Autodesk Inventor part; units mm, degrees
(part 10 of 13)
  arc A3550 (1.0789, 34.461) -> (1.0789, 34.335) centre (1.0789, 34.398) ccw
  line L3551 (3.0258, 34.335) -> (6.4346, 34.335)
  arc A3551 (6.4346, 34.335) -> (6.4346, 34.461) centre (6.4346, 34.398) ccw
  line L3552 (6.4346, 34.461) -> (3.0258, 34.461)
  arc A3552 (3.0258, 34.461) -> (3.0258, 34.335) centre (3.0258, 34.398) ccw
  line L3553 (8.9653, 34.335) -> (17.121, 34.335)
  arc A3553 (17.121, 34.335) -> (17.121, 34.461) centre (17.121, 34.398) ccw
  line L3554 (17.121, 34.461) -> (8.9653, 34.461)
  arc A3554 (8.9653, 34.461) -> (8.9653, 34.335) centre (8.9653, 34.398) ccw
  line L3555 (1.0789, 34.461) -> (2.0784, 34.461)
  arc A3555 (2.0784, 34.461) -> (2.0784, 34.587) centre (2.0784, 34.524) ccw
  line L3556 (2.0784, 34.587) -> (1.0789, 34.587)
  arc A3556 (1.0789, 34.587) -> (1.0789, 34.461) centre (1.0789, 34.524) ccw
  line L3557 (2.7216, 34.461) -> (6.4346, 34.461)
  arc A3557 (6.4346, 34.461) -> (6.4346, 34.587) centre (6.4346, 34.524) ccw
  line L3558 (6.4346, 34.587) -> (2.7216, 34.587)
  arc A3558 (2.7216, 34.587) -> (2.7216, 34.461) centre (2.7216, 34.524) ccw
  line L3559 (8.9653, 34.461) -> (17.121, 34.461)
  arc A3559 (17.121, 34.461) -> (17.121, 34.587) centre (17.121, 34.524) ccw
  line L3560 (17.121, 34.587) -> (8.9653, 34.587)
  arc A3560 (8.9653, 34.587) -> (8.9653, 34.461) centre (8.9653, 34.524) ccw
  line L3561 (1.0789, 34.587) -> (6.4346, 34.587)
  arc A3561 (6.4346, 34.587) -> (6.4346, 34.713) centre (6.4346, 34.65) ccw
  line L3562 (6.4346, 34.713) -> (1.0789, 34.713)
  arc A3562 (1.0789, 34.713) -> (1.0789, 34.587) centre (1.0789, 34.65) ccw
  line L3563 (8.9653, 34.587) -> (17.121, 34.587)
  arc A3563 (17.121, 34.587) -> (17.121, 34.713) centre (17.121, 34.65) ccw
  line L3564 (17.121, 34.713) -> (8.9653, 34.713)
  arc A3564 (8.9653, 34.713) -> (8.9653, 34.587) centre (8.9653, 34.65) ccw
  line L3565 (1.0789, 34.713) -> (6.4346, 34.713)
  arc A3565 (6.4346, 34.713) -> (6.4346, 34.839) centre (6.4346, 34.776) ccw
  line L3566 (6.4346, 34.839) -> (1.0789, 34.839)
  arc A3566 (1.0789, 34.839) -> (1.0789, 34.713) centre (1.0789, 34.776) ccw
  line L3567 (8.9653, 34.713) -> (17.121, 34.713)
  arc A3567 (17.121, 34.713) -> (17.121, 34.839) centre (17.121, 34.776) ccw
  line L3568 (17.121, 34.839) -> (8.9653, 34.839)
  arc A3568 (8.9653, 34.839) -> (8.9653, 34.713) centre (8.9653, 34.776) ccw
  line L3569 (1.0789, 34.839) -> (6.4803, 34.839)
  arc A3569 (6.4803, 34.839) -> (6.4803, 34.965) centre (6.4803, 34.902) ccw
  line L3570 (6.4803, 34.965) -> (1.0789, 34.965)
  arc A3570 (1.0789, 34.965) -> (1.0789, 34.839) centre (1.0789, 34.902) ccw
  line L3571 (8.9197, 34.839) -> (17.121, 34.839)
  arc A3571 (17.121, 34.839) -> (17.121, 34.965) centre (17.121, 34.902) ccw
  line L3572 (17.121, 34.965) -> (8.9197, 34.965)
  arc A3572 (8.9197, 34.965) -> (8.9197, 34.839) centre (8.9197, 34.902) ccw
  line L3573 (1.0789, 34.965) -> (6.5325, 34.965)
  arc A3573 (6.5325, 34.965) -> (6.5325, 35.091) centre (6.5325, 35.028) ccw
  line L3574 (6.5325, 35.091) -> (1.0789, 35.091)
  arc A3574 (1.0789, 35.091) -> (1.0789, 34.965) centre (1.0789, 35.028) ccw
  line L3575 (8.8675, 34.965) -> (17.121, 34.965)
  arc A3575 (17.121, 34.965) -> (17.121, 35.091) centre (17.121, 35.028) ccw
  line L3576 (17.121, 35.091) -> (8.8675, 35.091)
  arc A3576 (8.8675, 35.091) -> (8.8675, 34.965) centre (8.8675, 35.028) ccw
  line L3577 (1.0789, 35.091) -> (6.5847, 35.091)
  arc A3577 (6.5847, 35.091) -> (6.5847, 35.217) centre (6.5847, 35.154) ccw
  line L3578 (6.5847, 35.217) -> (1.0789, 35.217)
  arc A3578 (1.0789, 35.217) -> (1.0789, 35.091) centre (1.0789, 35.154) ccw
  line L3579 (8.8153, 35.091) -> (17.121, 35.091)
  arc A3579 (17.121, 35.091) -> (17.121, 35.217) centre (17.121, 35.154) ccw
  line L3580 (17.121, 35.217) -> (8.8153, 35.217)
  arc A3580 (8.8153, 35.217) -> (8.8153, 35.091) centre (8.8153, 35.154) ccw
  line L3581 (1.0789, 35.217) -> (6.6505, 35.217)
  arc A3581 (6.6505, 35.217) -> (6.6505, 35.343) centre (6.6505, 35.28) ccw
  line L3582 (6.6505, 35.343) -> (1.0789, 35.343)
  arc A3582 (1.0789, 35.343) -> (1.0789, 35.217) centre (1.0789, 35.28) ccw
  line L3583 (8.7494, 35.217) -> (17.121, 35.217)
  arc A3583 (17.121, 35.217) -> (17.121, 35.343) centre (17.121, 35.28) ccw
  line L3584 (17.121, 35.343) -> (8.7494, 35.343)
  arc A3584 (8.7494, 35.343) -> (8.7494, 35.217) centre (8.7494, 35.28) ccw
  line L3585 (1.0789, 35.343) -> (6.7765, 35.343)
  arc A3585 (6.7765, 35.343) -> (6.7765, 35.469) centre (6.7765, 35.406) ccw
  line L3586 (6.7765, 35.469) -> (1.0789, 35.469)
  arc A3586 (1.0789, 35.469) -> (1.0789, 35.343) centre (1.0789, 35.406) ccw
  line L3587 (8.6234, 35.343) -> (17.121, 35.343)
  arc A3587 (17.121, 35.343) -> (17.121, 35.469) centre (17.121, 35.406) ccw
  line L3588 (17.121, 35.469) -> (8.6234, 35.469)
  arc A3588 (8.6234, 35.469) -> (8.6234, 35.343) centre (8.6234, 35.406) ccw
  line L3589 (1.0789, 35.469) -> (6.9025, 35.469)
  arc A3589 (6.9025, 35.469) -> (6.9025, 35.595) centre (6.9025, 35.532) ccw
  line L3590 (6.9025, 35.595) -> (1.0789, 35.595)
  arc A3590 (1.0789, 35.595) -> (1.0789, 35.469) centre (1.0789, 35.532) ccw
  line L3591 (8.4974, 35.469) -> (17.121, 35.469)
  arc A3591 (17.121, 35.469) -> (17.121, 35.595) centre (17.121, 35.532) ccw
  line L3592 (17.121, 35.595) -> (8.4974, 35.595)
  arc A3592 (8.4974, 35.595) -> (8.4974, 35.469) centre (8.4974, 35.532) ccw
  line L3593 (1.0789, 35.595) -> (7.0926, 35.595)
  arc A3593 (7.0926, 35.595) -> (7.0926, 35.721) centre (7.0926, 35.658) ccw
  line L3594 (7.0926, 35.721) -> (1.0789, 35.721)
  arc A3594 (1.0789, 35.721) -> (1.0789, 35.595) centre (1.0789, 35.658) ccw
  line L3595 (8.3074, 35.595) -> (17.121, 35.595)
  arc A3595 (17.121, 35.595) -> (17.121, 35.721) centre (17.121, 35.658) ccw
  line L3596 (17.121, 35.721) -> (8.3074, 35.721)
  arc A3596 (8.3074, 35.721) -> (8.3074, 35.595) centre (8.3074, 35.658) ccw
  line L3597 (1.0789, 35.721) -> (2.0347, 35.721)
  arc A3597 (2.0347, 35.721) -> (2.0347, 35.847) centre (2.0347, 35.784) ccw
  line L3598 (2.0347, 35.847) -> (1.0789, 35.847)
  arc A3598 (1.0789, 35.847) -> (1.0789, 35.721) centre (1.0789, 35.784) ccw
  line L3599 (2.337, 35.721) -> (2.4628, 35.721)
  arc A3599 (2.4628, 35.721) -> (2.4628, 35.847) centre (2.4628, 35.784) ccw
  line L3600 (2.4628, 35.847) -> (2.337, 35.847)
  arc A3600 (2.337, 35.847) -> (2.337, 35.721) centre (2.337, 35.784) ccw
  line L3601 (2.7651, 35.721) -> (7.3968, 35.721)
  arc A3601 (7.3968, 35.721) -> (7.3968, 35.847) centre (7.3968, 35.784) ccw
  line L3602 (7.3968, 35.847) -> (2.7651, 35.847)
  arc A3602 (2.7651, 35.847) -> (2.7651, 35.721) centre (2.7651, 35.784) ccw
  line L3603 (8.0032, 35.721) -> (17.121, 35.721)
  arc A3603 (17.121, 35.721) -> (17.121, 35.847) centre (17.121, 35.784) ccw
  line L3604 (17.121, 35.847) -> (8.0032, 35.847)
  arc A3604 (8.0032, 35.847) -> (8.0032, 35.721) centre (8.0032, 35.784) ccw
  line L3605 (1.0789, 35.847) -> (1.7306, 35.847)
  arc A3605 (1.7306, 35.847) -> (1.7306, 35.973) centre (1.7306, 35.91) ccw
  line L3606 (1.7306, 35.973) -> (1.0789, 35.973)
  arc A3606 (1.0789, 35.973) -> (1.0789, 35.847) centre (1.0789, 35.91) ccw
  line L3607 (2.337, 35.847) -> (2.4628, 35.847)
  arc A3607 (2.4628, 35.847) -> (2.4628, 35.973) centre (2.4628, 35.91) ccw
  line L3608 (2.4628, 35.973) -> (2.337, 35.973)
  arc A3608 (2.337, 35.973) -> (2.337, 35.847) centre (2.337, 35.91) ccw
  line L3609 (3.0692, 35.847) -> (17.121, 35.847)
  arc A3609 (17.121, 35.847) -> (17.121, 35.973) centre (17.121, 35.91) ccw
  line L3610 (17.121, 35.973) -> (3.0692, 35.973)
  arc A3610 (3.0692, 35.973) -> (3.0692, 35.847) centre (3.0692, 35.91) ccw
  line L3611 (1.0789, 35.973) -> (1.5929, 35.973)
  arc A3611 (1.5929, 35.973) -> (1.5929, 36.099) centre (1.5929, 36.036) ccw
  line L3612 (1.5929, 36.099) -> (1.0789, 36.099)
  arc A3612 (1.0789, 36.099) -> (1.0789, 35.973) centre (1.0789, 36.036) ccw
  line L3613 (2.337, 35.973) -> (2.4628, 35.973)
  arc A3613 (2.4628, 35.973) -> (2.4628, 36.099) centre (2.4628, 36.036) ccw
  line L3614 (2.4628, 36.099) -> (2.337, 36.099)
  arc A3614 (2.337, 36.099) -> (2.337, 35.973) centre (2.337, 36.036) ccw
  line L3615 (3.207, 35.973) -> (17.121, 35.973)
  arc A3615 (17.121, 35.973) -> (17.121, 36.099) centre (17.121, 36.036) ccw
  line L3616 (17.121, 36.099) -> (3.207, 36.099)
  arc A3616 (3.207, 36.099) -> (3.207, 35.973) centre (3.207, 36.036) ccw
  line L3617 (1.0789, 36.099) -> (1.4669, 36.099)
  arc A3617 (1.4669, 36.099) -> (1.4669, 36.225) centre (1.4669, 36.162) ccw
  line L3618 (1.4669, 36.225) -> (1.0789, 36.225)
  arc A3618 (1.0789, 36.225) -> (1.0789, 36.099) centre (1.0789, 36.162) ccw
  line L3619 (2.337, 36.099) -> (2.4628, 36.099)
  arc A3619 (2.4628, 36.099) -> (2.4628, 36.225) centre (2.4628, 36.162) ccw
  line L3620 (2.4628, 36.225) -> (2.337, 36.225)
  arc A3620 (2.337, 36.225) -> (2.337, 36.099) centre (2.337, 36.162) ccw
  line L3621 (3.333, 36.099) -> (17.121, 36.099)
  arc A3621 (17.121, 36.099) -> (17.121, 36.225) centre (17.121, 36.162) ccw
  line L3622 (17.121, 36.225) -> (3.333, 36.225)
  arc A3622 (3.333, 36.225) -> (3.333, 36.099) centre (3.333, 36.162) ccw
  line L3623 (1.0789, 36.225) -> (1.3569, 36.225)
  arc A3623 (1.3569, 36.225) -> (1.3569, 36.351) centre (1.3569, 36.288) ccw
  line L3624 (1.3569, 36.351) -> (1.0789, 36.351)
  arc A3624 (1.0789, 36.351) -> (1.0789, 36.225) centre (1.0789, 36.288) ccw
  line L3625 (2.337, 36.225) -> (2.4628, 36.225)
  arc A3625 (2.4628, 36.225) -> (2.4628, 36.351) centre (2.4628, 36.288) ccw
  line L3626 (2.4628, 36.351) -> (2.337, 36.351)
  arc A3626 (2.337, 36.351) -> (2.337, 36.225) centre (2.337, 36.288) ccw
  line L3627 (3.4429, 36.225) -> (17.121, 36.225)
  arc A3627 (17.121, 36.225) -> (17.121, 36.351) centre (17.121, 36.288) ccw
  line L3628 (17.121, 36.351) -> (3.4429, 36.351)
  arc A3628 (3.4429, 36.351) -> (3.4429, 36.225) centre (3.4429, 36.288) ccw
  line L3629 (1.0789, 36.351) -> (1.3047, 36.351)
  arc A3629 (1.3047, 36.351) -> (1.3047, 36.477) centre (1.3047, 36.414) ccw
  line L3630 (1.3047, 36.477) -> (1.0789, 36.477)
  arc A3630 (1.0789, 36.477) -> (1.0789, 36.351) centre (1.0789, 36.414) ccw
  line L3631 (2.337, 36.351) -> (2.4628, 36.351)
  arc A3631 (2.4628, 36.351) -> (2.4628, 36.477) centre (2.4628, 36.414) ccw
  line L3632 (2.4628, 36.477) -> (2.337, 36.477)
  arc A3632 (2.337, 36.477) -> (2.337, 36.351) centre (2.337, 36.414) ccw
  line L3633 (3.4951, 36.351) -> (17.121, 36.351)
  arc A3633 (17.121, 36.351) -> (17.121, 36.477) centre (17.121, 36.414) ccw
  line L3634 (17.121, 36.477) -> (3.4951, 36.477)
  arc A3634 (3.4951, 36.477) -> (3.4951, 36.351) centre (3.4951, 36.414) ccw
  line L3635 (1.0789, 36.477) -> (1.2525, 36.477)
  arc A3635 (1.2525, 36.477) -> (1.2525, 36.603) centre (1.2525, 36.54) ccw
  line L3636 (1.2525, 36.603) -> (1.0789, 36.603)
  arc A3636 (1.0789, 36.603) -> (1.0789, 36.477) centre (1.0789, 36.54) ccw
  line L3637 (2.337, 36.477) -> (2.4628, 36.477)
  arc A3637 (2.4628, 36.477) -> (2.4628, 36.603) centre (2.4628, 36.54) ccw
  line L3638 (2.4628, 36.603) -> (2.337, 36.603)
  arc A3638 (2.337, 36.603) -> (2.337, 36.477) centre (2.337, 36.54) ccw
  line L3639 (3.5473, 36.477) -> (17.121, 36.477)
  arc A3639 (17.121, 36.477) -> (17.121, 36.603) centre (17.121, 36.54) ccw
  line L3640 (17.121, 36.603) -> (3.5473, 36.603)
  arc A3640 (3.5473, 36.603) -> (3.5473, 36.477) centre (3.5473, 36.54) ccw
  line L3641 (1.0789, 36.603) -> (1.2003, 36.603)
  arc A3641 (1.2003, 36.603) -> (1.2003, 36.729) centre (1.2003, 36.666) ccw
  line L3642 (1.2003, 36.729) -> (1.0789, 36.729)
  arc A3642 (1.0789, 36.729) -> (1.0789, 36.603) centre (1.0789, 36.666) ccw
  line L3643 (2.337, 36.603) -> (2.4628, 36.603)
  arc A3643 (2.4628, 36.603) -> (2.4628, 36.729) centre (2.4628, 36.666) ccw
  line L3644 (2.4628, 36.729) -> (2.337, 36.729)
  arc A3644 (2.337, 36.729) -> (2.337, 36.603) centre (2.337, 36.666) ccw
  line L3645 (3.5995, 36.603) -> (17.121, 36.603)
  arc A3645 (17.121, 36.603) -> (17.121, 36.729) centre (17.121, 36.666) ccw
  line L3646 (17.121, 36.729) -> (3.5995, 36.729)
  arc A3646 (3.5995, 36.729) -> (3.5995, 36.603) centre (3.5995, 36.666) ccw
  line L3647 (1.0789, 36.729) -> (1.183, 36.729)
  arc A3647 (1.183, 36.729) -> (1.183, 36.855) centre (1.183, 36.792) ccw
  line L3648 (1.183, 36.855) -> (1.0789, 36.855)
  arc A3648 (1.0789, 36.855) -> (1.0789, 36.729) centre (1.0789, 36.792) ccw
  line L3649 (2.337, 36.729) -> (2.4628, 36.729)
  arc A3649 (2.4628, 36.729) -> (2.4628, 36.855) centre (2.4628, 36.792) ccw
  line L3650 (2.4628, 36.855) -> (2.337, 36.855)
  arc A3650 (2.337, 36.855) -> (2.337, 36.729) centre (2.337, 36.792) ccw
  line L3651 (3.6169, 36.729) -> (17.121, 36.729)
  arc A3651 (17.121, 36.729) -> (17.121, 36.855) centre (17.121, 36.792) ccw
  line L3652 (17.121, 36.855) -> (3.6169, 36.855)
  arc A3652 (3.6169, 36.855) -> (3.6169, 36.729) centre (3.6169, 36.792) ccw
  line L3653 (1.0789, 36.855) -> (2.3365, 36.855)
  arc A3653 (2.3365, 36.855) -> (2.3365, 36.981) centre (2.3365, 36.918) ccw
  line L3654 (2.3365, 36.981) -> (1.0789, 36.981)
  arc A3654 (1.0789, 36.981) -> (1.0789, 36.855) centre (1.0789, 36.918) ccw
  line L3655 (2.4634, 36.855) -> (17.121, 36.855)
  arc A3655 (17.121, 36.855) -> (17.121, 36.981) centre (17.121, 36.918) ccw
  line L3656 (17.121, 36.981) -> (2.4634, 36.981)
  arc A3656 (2.4634, 36.981) -> (2.4634, 36.855) centre (2.4634, 36.918) ccw
  line L3657 (1.0789, 36.981) -> (1.183, 36.981)
  arc A3657 (1.183, 36.981) -> (1.183, 37.107) centre (1.183, 37.044) ccw
  line L3658 (1.183, 37.107) -> (1.0789, 37.107)
  arc A3658 (1.0789, 37.107) -> (1.0789, 36.981) centre (1.0789, 37.044) ccw
  line L3659 (2.337, 36.981) -> (2.4628, 36.981)
  arc A3659 (2.4628, 36.981) -> (2.4628, 37.107) centre (2.4628, 37.044) ccw
  line L3660 (2.4628, 37.107) -> (2.337, 37.107)
  arc A3660 (2.337, 37.107) -> (2.337, 36.981) centre (2.337, 37.044) ccw
  line L3661 (3.6169, 36.981) -> (17.121, 36.981)
  arc A3661 (17.121, 36.981) -> (17.121, 37.107) centre (17.121, 37.044) ccw
  line L3662 (17.121, 37.107) -> (3.6169, 37.107)
  arc A3662 (3.6169, 37.107) -> (3.6169, 36.981) centre (3.6169, 37.044) ccw
  line L3663 (1.0789, 37.107) -> (1.183, 37.107)
  arc A3663 (1.183, 37.107) -> (1.183, 37.233) centre (1.183, 37.17) ccw
  line L3664 (1.183, 37.233) -> (1.0789, 37.233)
  arc A3664 (1.0789, 37.233) -> (1.0789, 37.107) centre (1.0789, 37.17) ccw
  line L3665 (2.337, 37.107) -> (2.4628, 37.107)
  arc A3665 (2.4628, 37.107) -> (2.4628, 37.233) centre (2.4628, 37.17) ccw
  line L3666 (2.4628, 37.233) -> (2.337, 37.233)
  arc A3666 (2.337, 37.233) -> (2.337, 37.107) centre (2.337, 37.17) ccw
  line L3667 (3.6169, 37.107) -> (17.121, 37.107)
  arc A3667 (17.121, 37.107) -> (17.121, 37.233) centre (17.121, 37.17) ccw
  line L3668 (17.121, 37.233) -> (3.6169, 37.233)
  arc A3668 (3.6169, 37.233) -> (3.6169, 37.107) centre (3.6169, 37.17) ccw
  line L3669 (1.0789, 37.233) -> (1.2261, 37.233)
  arc A3669 (1.2261, 37.233) -> (1.2261, 37.359) centre (1.2261, 37.296) ccw
  line L3670 (1.2261, 37.359) -> (1.0789, 37.359)
  arc A3670 (1.0789, 37.359) -> (1.0789, 37.233) centre (1.0789, 37.296) ccw
  line L3671 (2.337, 37.233) -> (2.4628, 37.233)
  arc A3671 (2.4628, 37.233) -> (2.4628, 37.359) centre (2.4628, 37.296) ccw
  line L3672 (2.4628, 37.359) -> (2.337, 37.359)
  arc A3672 (2.337, 37.359) -> (2.337, 37.233) centre (2.337, 37.296) ccw
  line L3673 (3.5739, 37.233) -> (17.121, 37.233)
  arc A3673 (17.121, 37.233) -> (17.121, 37.359) centre (17.121, 37.296) ccw
  line L3674 (17.121, 37.359) -> (3.5739, 37.359)
  arc A3674 (3.5739, 37.359) -> (3.5739, 37.233) centre (3.5739, 37.296) ccw
  line L3675 (1.0789, 37.359) -> (1.2783, 37.359)
  arc A3675 (1.2783, 37.359) -> (1.2783, 37.485) centre (1.2783, 37.422) ccw
  line L3676 (1.2783, 37.485) -> (1.0789, 37.485)
  arc A3676 (1.0789, 37.485) -> (1.0789, 37.359) centre (1.0789, 37.422) ccw
  line L3677 (2.337, 37.359) -> (2.4628, 37.359)
  arc A3677 (2.4628, 37.359) -> (2.4628, 37.485) centre (2.4628, 37.422) ccw
  line L3678 (2.4628, 37.485) -> (2.337, 37.485)
  arc A3678 (2.337, 37.485) -> (2.337, 37.359) centre (2.337, 37.422) ccw
  line L3679 (3.5217, 37.359) -> (17.121, 37.359)
  arc A3679 (17.121, 37.359) -> (17.121, 37.485) centre (17.121, 37.422) ccw
  line L3680 (17.121, 37.485) -> (3.5217, 37.485)
  arc A3680 (3.5217, 37.485) -> (3.5217, 37.359) centre (3.5217, 37.422) ccw
  line L3681 (1.0789, 37.485) -> (1.3305, 37.485)
  arc A3681 (1.3305, 37.485) -> (1.3305, 37.611) centre (1.3305, 37.548) ccw
  line L3682 (1.3305, 37.611) -> (1.0789, 37.611)
  arc A3682 (1.0789, 37.611) -> (1.0789, 37.485) centre (1.0789, 37.548) ccw
  line L3683 (2.337, 37.485) -> (2.4628, 37.485)
  arc A3683 (2.4628, 37.485) -> (2.4628, 37.611) centre (2.4628, 37.548) ccw
  line L3684 (2.4628, 37.611) -> (2.337, 37.611)
  arc A3684 (2.337, 37.611) -> (2.337, 37.485) centre (2.337, 37.548) ccw
  line L3685 (3.4695, 37.485) -> (17.121, 37.485)
  arc A3685 (17.121, 37.485) -> (17.121, 37.611) centre (17.121, 37.548) ccw
  line L3686 (17.121, 37.611) -> (3.4695, 37.611)
  arc A3686 (3.4695, 37.611) -> (3.4695, 37.485) centre (3.4695, 37.548) ccw
  line L3687 (1.0789, 37.611) -> (1.403, 37.611)
  arc A3687 (1.403, 37.611) -> (1.403, 37.737) centre (1.403, 37.674) ccw
  line L3688 (1.403, 37.737) -> (1.0789, 37.737)
  arc A3688 (1.0789, 37.737) -> (1.0789, 37.611) centre (1.0789, 37.674) ccw
  line L3689 (2.337, 37.611) -> (2.4628, 37.611)
  arc A3689 (2.4628, 37.611) -> (2.4628, 37.737) centre (2.4628, 37.674) ccw
  line L3690 (2.4628, 37.737) -> (2.337, 37.737)
  arc A3690 (2.337, 37.737) -> (2.337, 37.611) centre (2.337, 37.674) ccw
  line L3691 (3.3969, 37.611) -> (17.121, 37.611)
  arc A3691 (17.121, 37.611) -> (17.121, 37.737) centre (17.121, 37.674) ccw
  line L3692 (17.121, 37.737) -> (3.3969, 37.737)
  arc A3692 (3.3969, 37.737) -> (3.3969, 37.611) centre (3.3969, 37.674) ccw
  line L3693 (1.0789, 37.737) -> (1.529, 37.737)
  arc A3693 (1.529, 37.737) -> (1.529, 37.863) centre (1.529, 37.8) ccw
  line L3694 (1.529, 37.863) -> (1.0789, 37.863)
  arc A3694 (1.0789, 37.863) -> (1.0789, 37.737) centre (1.0789, 37.8) ccw
  line L3695 (2.337, 37.737) -> (2.4628, 37.737)
  arc A3695 (2.4628, 37.737) -> (2.4628, 37.863) centre (2.4628, 37.8) ccw
  line L3696 (2.4628, 37.863) -> (2.337, 37.863)
  arc A3696 (2.337, 37.863) -> (2.337, 37.737) centre (2.337, 37.8) ccw
  line L3697 (3.2709, 37.737) -> (17.121, 37.737)
  arc A3697 (17.121, 37.737) -> (17.121, 37.863) centre (17.121, 37.8) ccw
  line L3698 (17.121, 37.863) -> (3.2709, 37.863)
  arc A3698 (3.2709, 37.863) -> (3.2709, 37.737) centre (3.2709, 37.8) ccw
  line L3699 (1.0789, 37.863) -> (1.655, 37.863)
  arc A3699 (1.655, 37.863) -> (1.655, 37.989) centre (1.655, 37.926) ccw
  line L3700 (1.655, 37.989) -> (1.0789, 37.989)
  arc A3700 (1.0789, 37.989) -> (1.0789, 37.863) centre (1.0789, 37.926) ccw
  line L3701 (2.337, 37.863) -> (2.4628, 37.863)
  arc A3701 (2.4628, 37.863) -> (2.4628, 37.989) centre (2.4628, 37.926) ccw
  line L3702 (2.4628, 37.989) -> (2.337, 37.989)
  arc A3702 (2.337, 37.989) -> (2.337, 37.863) centre (2.337, 37.926) ccw
  line L3703 (3.1449, 37.863) -> (17.121, 37.863)
  arc A3703 (17.121, 37.863) -> (17.121, 37.989) centre (17.121, 37.926) ccw
  line L3704 (17.121, 37.989) -> (3.1449, 37.989)
  arc A3704 (3.1449, 37.989) -> (3.1449, 37.863) centre (3.1449, 37.926) ccw
  line L3705 (1.0789, 37.989) -> (1.8806, 37.989)
  arc A3705 (1.8806, 37.989) -> (1.8806, 38.115) centre (1.8806, 38.052) ccw
  line L3706 (1.8806, 38.115) -> (1.0789, 38.115)
  arc A3706 (1.0789, 38.115) -> (1.0789, 37.989) centre (1.0789, 38.052) ccw
  line L3707 (2.337, 37.989) -> (2.4628, 37.989)
  arc A3707 (2.4628, 37.989) -> (2.4628, 38.115) centre (2.4628, 38.052) ccw
  line L3708 (2.4628, 38.115) -> (2.337, 38.115)
  arc A3708 (2.337, 38.115) -> (2.337, 37.989) centre (2.337, 38.052) ccw
  line L3709 (2.9194, 37.989) -> (17.121, 37.989)
  arc A3709 (17.121, 37.989) -> (17.121, 38.115) centre (17.121, 38.052) ccw
  line L3710 (17.121, 38.115) -> (2.9194, 38.115)
  arc A3710 (2.9194, 38.115) -> (2.9194, 37.989) centre (2.9194, 38.052) ccw
  line L3711 (1.0789, 38.115) -> (17.121, 38.115)
  arc A3711 (17.121, 38.115) -> (17.121, 38.241) centre (17.121, 38.178) ccw
  line L3712 (17.121, 38.241) -> (1.0789, 38.241)
  arc A3712 (1.0789, 38.241) -> (1.0789, 38.115) centre (1.0789, 38.178) ccw
  line L3713 (1.0789, 38.241) -> (7.3048, 38.241)
  arc A3713 (7.3048, 38.241) -> (7.3048, 38.367) centre (7.3048, 38.304) ccw
  line L3714 (7.3048, 38.367) -> (1.0789, 38.367)
  arc A3714 (1.0789, 38.367) -> (1.0789, 38.241) centre (1.0789, 38.304) ccw
  line L3715 (7.637, 38.241) -> (7.7628, 38.241)
  arc A3715 (7.7628, 38.241) -> (7.7628, 38.367) centre (7.7628, 38.304) ccw
  line L3716 (7.7628, 38.367) -> (7.637, 38.367)
  arc A3716 (7.637, 38.367) -> (7.637, 38.241) centre (7.637, 38.304) ccw
  line L3717 (8.095, 38.241) -> (17.121, 38.241)
  arc A3717 (17.121, 38.241) -> (17.121, 38.367) centre (17.121, 38.304) ccw
  arc A3718 (6.9929, 25.0871) -> (8.4071, 23.6729) centre (7.7, 24.38) ccw
  line L3718 (2.4, 39.45) -> (3.75, 39.45)
  arc A3719 (3.75, 39.45) -> (3.75, 41.45) centre (3.75, 40.45) ccw
  line L3719 (3.75, 41.45) -> (2.4, 41.45)
  arc A3720 (2.4, 41.45) -> (2.4, 39.45) centre (2.4, 40.45) ccw
  line L3720 (3.0429, 39.7429) -> (4.2929, 38.4929)
  arc A3721 (4.2929, 38.4929) -> (5.7071, 39.9071) centre (5, 39.2) ccw
  arc A3722 (6.5829, 55.1571) -> (7.9971, 53.7429) centre (7.29, 54.45) ccw
  line L3721 (5.7071, 39.9071) -> (4.4571, 41.1571)
  arc A3723 (4.4571, 41.1571) -> (3.0429, 39.7429) centre (3.75, 40.45) ccw
  line L3722 (4, 39.2) -> (4, 37.24)
  arc A3724 (4, 37.24) -> (6, 37.24) centre (5, 37.24) ccw
  line L3723 (6, 37.24) -> (6, 39.2)
  arc A3725 (6, 39.2) -> (4, 39.2) centre (5, 39.2) ccw
  arc A3726 (3.1071, 27.1571) -> (1.6929, 25.7429) centre (2.4, 26.45) ccw
  line L3724 (4.2929, 36.5329) -> (6.9929, 33.8329)
  arc A3727 (6.9929, 33.8329) -> (8.4071, 35.2471) centre (7.7, 34.54) ccw
  line L3725 (8.4071, 35.2471) -> (5.7071, 37.9471)
  arc A3728 (5.7071, 37.9471) -> (4.2929, 36.5329) centre (5, 37.24) ccw
  arc A3729 (4.95, 46.45) -> (4.95, 48.45) centre (4.95, 47.45) ccw
  line L3726 (4.95, 48.45) -> (2.4, 48.45)
  arc A3730 (2.4, 48.45) -> (2.4, 46.45) centre (2.4, 47.45) ccw
  line L3727 (4.2429, 46.7429) -> (6.9929, 43.9929)
  arc A3731 (6.9929, 43.9929) -> (8.4071, 45.4071) centre (7.7, 44.7) ccw
  line L3728 (8.4071, 45.4071) -> (5.6571, 48.1571)
  arc A3732 (5.6571, 48.1571) -> (4.2429, 46.7429) centre (4.95, 47.45) ccw
  line L3729 (2.4, 53.45) -> (7.29, 53.45)
  arc A3733 (7.29, 53.45) -> (7.29, 55.45) centre (7.29, 54.45) ccw
  line L3730 (7.29, 55.45) -> (2.4, 55.45)
  arc A3734 (2.4, 55.45) -> (2.4, 53.45) centre (2.4, 54.45) ccw
  line L3731 (7.9971, 53.7429) -> (8.4071, 54.1529)
  arc A3735 (8.4071, 54.1529) -> (6.9929, 55.5671) centre (7.7, 54.86) ccw
  line L3732 (6.9929, 55.5671) -> (6.5829, 55.1571)
  line L3733 (4.74, 3.06) -> (7.7, 3.06)
  arc A3736 (7.7, 3.06) -> (7.7, 5.06) centre (7.7, 4.06) ccw
  line L3734 (7.7, 5.06) -> (4.74, 5.06)
  arc A3737 (4.74, 5.06) -> (4.74, 3.06) centre (4.74, 4.06) ccw
  line L3735 (1.6929, 5.6929) -> (4.0329, 3.3529)
  arc A3738 (4.0329, 3.3529) -> (5.4471, 4.7671) centre (4.74, 4.06) ccw
  line L3736 (5.4471, 4.7671) -> (3.1071, 7.1071)
  arc A3739 (3.1071, 7.1071) -> (1.6929, 5.6929) centre (2.4, 6.4) ccw
  line L3737 (3.4, 6.4) -> (3.4, 19.45)
  arc A3740 (3.4, 19.45) -> (1.4, 19.45) centre (2.4, 19.45) ccw
  line L3738 (1.4, 19.45) -> (1.4, 6.4)
  arc A3741 (1.4, 6.4) -> (3.4, 6.4) centre (2.4, 6.4) ccw
  line L3739 (7.38, 13.22) -> (7.7, 13.22)
  arc A3742 (7.7, 13.22) -> (7.7, 15.22) centre (7.7, 14.22) ccw
  line L3740 (7.7, 15.22) -> (7.38, 15.22)
  arc A3743 (7.38, 15.22) -> (7.38, 13.22) centre (7.38, 14.22) ccw
  line L3741 (8.0871, 14.9271) -> (6.1071, 16.9071)
  arc A3744 (6.1071, 16.9071) -> (4.6929, 15.4929) centre (5.4, 16.2) ccw
  line L3742 (4.6929, 15.4929) -> (6.6729, 13.5129)
  arc A3745 (6.6729, 13.5129) -> (8.0871, 14.9271) centre (7.38, 14.22) ccw
  line L3743 (6.4, 16.2) -> (6.4, 23.45)
  arc A3746 (6.4, 23.45) -> (4.4, 23.45) centre (5.4, 23.45) ccw
  line L3744 (4.4, 23.45) -> (4.4, 16.2)
  arc A3747 (4.4, 16.2) -> (6.4, 16.2) centre (5.4, 16.2) ccw
  line L3745 (6.1071, 24.1571) -> (3.1071, 27.1571)
  line L3746 (2.4, 46.45) -> (4.95, 46.45)
  line L3747 (1.6929, 25.7429) -> (4.6929, 22.7429)
  arc A3748 (4.6929, 22.7429) -> (6.1071, 24.1571) centre (5.4, 23.45) ccw
  line L3748 (3.35, 34.45) -> (2.4, 34.45)
  arc A3749 (2.4, 34.45) -> (2.4, 32.45) centre (2.4, 33.45) ccw
  line L3749 (2.4, 32.45) -> (3.35, 32.45)
  arc A3750 (3.35, 32.45) -> (3.35, 34.45) centre (3.35, 33.45) ccw
  line L3750 (5.5071, 32.7071) -> (4.0571, 34.1571)
  arc A3751 (4.0571, 34.1571) -> (2.6429, 32.7429) centre (3.35, 33.45) ccw
  line L3751 (2.6429, 32.7429) -> (4.0929, 31.2929)
  arc A3752 (4.0929, 31.2929) -> (5.5071, 32.7071) centre (4.8, 32) ccw
  line L3752 (8.8, 33) -> (4.8, 33)
  arc A3753 (4.8, 33) -> (4.8, 31) centre (4.8, 32) ccw
  line L3753 (4.8, 31) -> (8.8, 31)
  arc A3754 (8.8, 31) -> (8.8, 33) centre (8.8, 32) ccw
  line L3754 (11.3071, 30.9071) -> (9.5071, 32.7071)
  arc A3755 (9.5071, 32.7071) -> (8.0929, 31.2929) centre (8.8, 32) ccw
  line L3755 (8.0929, 31.2929) -> (9.8929, 29.4929)
  arc A3756 (9.8929, 29.4929) -> (11.3071, 30.9071) centre (10.6, 30.2) ccw
  line L3756 (11.6, 27.28) -> (11.6, 30.2)
  arc A3757 (11.6, 30.2) -> (9.6, 30.2) centre (10.6, 30.2) ccw
  line L3757 (9.6, 30.2) -> (9.6, 27.28)
  arc A3758 (9.6, 27.28) -> (11.6, 27.28) centre (10.6, 27.28) ccw
  line L3758 (8.4071, 23.6729) -> (11.3071, 26.5729)
  arc A3759 (11.3071, 26.5729) -> (9.8929, 27.9871) centre (10.6, 27.28) ccw
  line L3759 (9.8929, 27.9871) -> (6.9929, 25.0871)
  line L3760 (0, 0) -> (18.2, 0)
  line L3761 (18.2, 0) -> (18.2, 64.3)
  line L3762 (18.2, 64.3) -> (0, 64.3)
  line L3763 (0, 64.3) -> (0, 0)
  line L3764 (0.5865, 59.7) -> (0.5865, 17.7)
  arc A3760 (0.7135, 59.7) -> (0.5865, 59.7) centre (0.65, 59.7) ccw
  line L3765 (0.7135, 17.7) -> (0.7135, 59.7)
  arc A3761 (0.5865, 17.7) -> (0.7135, 17.7) centre (0.65, 17.7) ccw
  line L3766 (0.65, 59.6365) -> (4.15, 59.6365)
  arc A3762 (4.15, 59.6365) -> (4.15, 59.7635) centre (4.15, 59.7) ccw
  line L3767 (4.15, 59.7635) -> (0.65, 59.7635)
  arc A3763 (0.65, 59.7635) -> (0.65, 59.6365) centre (0.65, 59.7) ccw
  line L3768 (4.0865, 59.7) -> (4.0865, 17.7)
  line L3769 (4.2135, 17.7) -> (4.2135, 59.7)
  arc A3764 (4.2135, 59.7) -> (4.0865, 59.7) centre (4.15, 59.7) ccw
  line L3770 (4.15, 17.7635) -> (0.65, 17.7635)
  arc A3765 (0.65, 17.7635) -> (0.65, 17.6365) centre (0.65, 17.7) ccw
  line L3771 (0.65, 17.6365) -> (4.15, 17.6365)
  arc A3766 (4.15, 17.6365) -> (4.15, 17.7635) centre (4.15, 17.7) ccw
  line L3772 (17.86, 0.3135) -> (5.16, 0.3135)
  arc A3767 (5.16, 0.3135) -> (5.16, 0.1865) centre (5.16, 0.25) ccw
  line L3773 (5.16, 0.1865) -> (17.86, 0.1865)
  arc A3768 (17.86, 0.1865) -> (17.86, 0.3135) centre (17.86, 0.25) ccw
  line L3774 (5.2235, 0.25) -> (5.2235, 63.75)
  arc A3769 (5.2235, 63.75) -> (5.0965, 63.75) centre (5.16, 63.75) ccw
  line L3775 (5.0965, 63.75) -> (5.0965, 0.25)
  arc A3770 (5.0965, 0.25) -> (5.2235, 0.25) centre (5.16, 0.25) ccw
  line L3776 (5.16, 63.6865) -> (17.86, 63.6865)
  arc A3771 (17.86, 63.6865) -> (17.86, 63.8135) centre (17.86, 63.75) ccw
  line L3777 (17.86, 63.8135) -> (5.16, 63.8135)
  arc A3772 (5.16, 63.8135) -> (5.16, 63.6865) centre (5.16, 63.75) ccw
  arc A3773 (4.0865, 17.7) -> (4.2135, 17.7) centre (4.15, 17.7) ccw
  line L3778 (16.5247, 5.1578) -> (15.4062, 5.1578)
  arc A3774 (15.4062, 5.1578) -> (15.4062, 5.0054) centre (15.4062, 5.0816) ccw
  line L3779 (15.4062, 5.0054) -> (16.5247, 5.0054)
  arc A3775 (16.5247, 5.0054) -> (16.5247, 5.1578) centre (16.5247, 5.0816) ccw
  line L3780 (15.4062, 5.429) -> (16.5247, 5.429)
  arc A3776 (16.5247, 5.429) -> (16.5247, 5.5814) centre (16.5247, 5.5052) ccw
  line L3781 (16.5247, 5.5814) -> (15.4062, 5.5814)
  arc A3777 (15.4062, 5.5814) -> (15.4062, 5.429) centre (15.4062, 5.5052) ccw
  line L3782 (16.5786, 5.5591) -> (16.2058, 5.9319)
  arc A3778 (16.2058, 5.9319) -> (16.098, 5.8241) centre (16.1519, 5.878) ccw
  line L3783 (16.098, 5.8241) -> (16.4708, 5.4513)
  arc A3779 (16.4708, 5.4513) -> (16.5786, 5.5591) centre (16.5247, 5.5052) ccw
  line L3784 (16.2058, 5.8241) -> (16.5786, 6.197)
  arc A3780 (16.5786, 6.197) -> (16.4708, 6.3048) centre (16.5247, 6.2509) ccw
  line L3785 (16.4708, 6.3048) -> (16.098, 5.9319)
  arc A3781 (16.098, 5.9319) -> (16.2058, 5.8241) centre (16.1519, 5.878) ccw
  line L3786 (16.5247, 6.3271) -> (15.4062, 6.3271)
  arc A3782 (15.4062, 6.3271) -> (15.4062, 6.1747) centre (15.4062, 6.2509) ccw
  line L3787 (15.4062, 6.1747) -> (16.5247, 6.1747)
  arc A3783 (16.5247, 6.1747) -> (16.5247, 6.3271) centre (16.5247, 6.2509) ccw
  line L3788 (16.0416, 6.6745) -> (16.0416, 7.4202)
  arc A3784 (16.0416, 7.4202) -> (15.8892, 7.4202) centre (15.9654, 7.4202) ccw
  line L3789 (15.8892, 7.4202) -> (15.8892, 6.6745)
  arc A3785 (15.8892, 6.6745) -> (16.0416, 6.6745) centre (15.9654, 6.6745) ccw
  line L3790 (16.4485, 8.5895) -> (16.4485, 7.8438)
  arc A3786 (16.4485, 7.8438) -> (16.6009, 7.8438) centre (16.5247, 7.8438) ccw
  line L3791 (16.6009, 7.8438) -> (16.6009, 8.5895)
  arc A3787 (16.6009, 8.5895) -> (16.4485, 8.5895) centre (16.5247, 8.5895) ccw
  line L3792 (16.5247, 7.92) -> (15.9654, 7.92)
  arc A3788 (15.9654, 7.92) -> (15.9654, 7.7676) centre (15.9654, 7.8438) ccw
  line L3793 (15.9654, 7.7676) -> (16.5247, 7.7676)
  arc A3789 (16.5247, 7.7676) -> (16.5247, 7.92) centre (16.5247, 7.8438) ccw
  line L3794 (16.0335, 7.8097) -> (16.22, 8.1825)
  arc A3790 (16.22, 8.1825) -> (16.0838, 8.2507) centre (16.1519, 8.2166) ccw
  line L3795 (16.0838, 8.2507) -> (15.8973, 7.8779)
  arc A3791 (15.8973, 7.8779) -> (16.0335, 7.8097) centre (15.9654, 7.8438) ccw
  line L3796 (16.2281, 8.2166) -> (16.2281, 8.403)
  arc A3792 (16.2281, 8.403) -> (16.0757, 8.403) centre (16.1519, 8.403) ccw
  line L3797 (16.0757, 8.403) -> (16.0757, 8.2166)
  arc A3793 (16.0757, 8.2166) -> (16.2281, 8.2166) centre (16.1519, 8.2166) ccw
  line L3798 (16.2058, 8.4569) -> (16.0193, 8.6434)
  arc A3794 (16.0193, 8.6434) -> (15.9115, 8.5356) centre (15.9654, 8.5895) ccw
  line L3799 (15.9115, 8.5356) -> (16.098, 8.3491)
  arc A3795 (16.098, 8.3491) -> (16.2058, 8.4569) centre (16.1519, 8.403) ccw
  line L3800 (15.9654, 8.6657) -> (15.5926, 8.6657)
  arc A3796 (15.5926, 8.6657) -> (15.5926, 8.5133) centre (15.5926, 8.5895) ccw
  line L3801 (15.5926, 8.5133) -> (15.9654, 8.5133)
  arc A3797 (15.9654, 8.5133) -> (15.9654, 8.6657) centre (15.9654, 8.5895) ccw
  line L3802 (15.5387, 8.6434) -> (15.3523, 8.4569)
  arc A3798 (15.3523, 8.4569) -> (15.4601, 8.3491) centre (15.4062, 8.403) ccw
  line L3803 (15.4601, 8.3491) -> (15.6465, 8.5356)
  arc A3799 (15.6465, 8.5356) -> (15.5387, 8.6434) centre (15.5926, 8.5895) ccw
  line L3804 (15.33, 8.403) -> (15.33, 8.0302)
  arc A3800 (15.33, 8.0302) -> (15.4824, 8.0302) centre (15.4062, 8.0302) ccw
  line L3805 (15.4824, 8.0302) -> (15.4824, 8.403)
  arc A3801 (15.4824, 8.403) -> (15.33, 8.403) centre (15.4062, 8.403) ccw
  line L3806 (15.3523, 7.9763) -> (15.5387, 7.7899)
  arc A3802 (15.5387, 7.7899) -> (15.6465, 7.8977) centre (15.5926, 7.8438) ccw
  line L3807 (15.6465, 7.8977) -> (15.4601, 8.0841)
  arc A3803 (15.4601, 8.0841) -> (15.3523, 7.9763) centre (15.4062, 8.0302) ccw
  line L3808 (15.4062, 8.9369) -> (15.5926, 8.9369)
  arc A3804 (15.5926, 8.9369) -> (15.5926, 9.0893) centre (15.5926, 9.0131) ccw
  line L3809 (15.5926, 9.0893) -> (15.4062, 9.0893)
  arc A3805 (15.4062, 9.0893) -> (15.4062, 8.9369) centre (15.4062, 9.0131) ccw
  line L3810 (15.6688, 9.0131) -> (15.6688, 9.1995)
  arc A3806 (15.6688, 9.1995) -> (15.5164, 9.1995) centre (15.5926, 9.1995) ccw
  line L3811 (15.5164, 9.1995) -> (15.5164, 9.0131)
  arc A3807 (15.5164, 9.0131) -> (15.6688, 9.0131) centre (15.5926, 9.0131) ccw
  line L3812 (15.5926, 9.2757) -> (15.4062, 9.2757)
  arc A3808 (15.4062, 9.2757) -> (15.4062, 9.1233) centre (15.4062, 9.1995) ccw
  line L3813 (15.4062, 9.1233) -> (15.5926, 9.1233)
  arc A3809 (15.5926, 9.1233) -> (15.5926, 9.2757) centre (15.5926, 9.1995) ccw
  line L3814 (15.33, 9.1995) -> (15.33, 9.0131)
  arc A3810 (15.33, 9.0131) -> (15.4824, 9.0131) centre (15.4062, 9.0131) ccw
  line L3815 (15.4824, 9.0131) -> (15.4824, 9.1995)
  arc A3811 (15.4824, 9.1995) -> (15.33, 9.1995) centre (15.4062, 9.1995) ccw
  line L3816 (15.5926, 9.5215) -> (16.3383, 9.5215)
  arc A3812 (16.3383, 9.5215) -> (16.3383, 9.6739) centre (16.3383, 9.5977) ccw
  line L3817 (16.3383, 9.6739) -> (15.5926, 9.6739)
  arc A3813 (15.5926, 9.6739) -> (15.5926, 9.5215) centre (15.5926, 9.5977) ccw
  line L3818 (16.3922, 9.5438) -> (16.5786, 9.7302)
  arc A3814 (16.5786, 9.7302) -> (16.4708, 9.838) centre (16.5247, 9.7841) ccw
  line L3819 (16.4708, 9.838) -> (16.2844, 9.6516)
  arc A3815 (16.2844, 9.6516) -> (16.3922, 9.5438) centre (16.3383, 9.5977) ccw
  line L3820 (16.6009, 9.7841) -> (16.6009, 10.1569)
  arc A3816 (16.6009, 10.1569) -> (16.4485, 10.1569) centre (16.5247, 10.1569) ccw
  line L3821 (16.4485, 10.1569) -> (16.4485, 9.7841)
  arc A3817 (16.4485, 9.7841) -> (16.6009, 9.7841) centre (16.5247, 9.7841) ccw
  line L3822 (16.5786, 10.2108) -> (16.3922, 10.3973)
  arc A3818 (16.3922, 10.3973) -> (16.2844, 10.2895) centre (16.3383, 10.3434) ccw
  line L3823 (16.2844, 10.2895) -> (16.4708, 10.103)
  arc A3819 (16.4708, 10.103) -> (16.5786, 10.2108) centre (16.5247, 10.1569) ccw
  line L3824 (16.3383, 10.4196) -> (15.5926, 10.4196)
  arc A3820 (15.5926, 10.4196) -> (15.5926, 10.2672) centre (15.5926, 10.3434) ccw
  line L3825 (15.5926, 10.2672) -> (16.3383, 10.2672)
  arc A3821 (16.3383, 10.2672) -> (16.3383, 10.4196) centre (16.3383, 10.3434) ccw
  line L3826 (15.5387, 10.3973) -> (15.3523, 10.2108)
  arc A3822 (15.3523, 10.2108) -> (15.4601, 10.103) centre (15.4062, 10.1569) ccw
  line L3827 (15.4601, 10.103) -> (15.6465, 10.2895)
  arc A3823 (15.6465, 10.2895) -> (15.5387, 10.3973) centre (15.5926, 10.3434) ccw
  line L3828 (15.33, 10.1569) -> (15.33, 9.7841)
  arc A3824 (15.33, 9.7841) -> (15.4824, 9.7841) centre (15.4062, 9.7841) ccw
  line L3829 (15.4824, 9.7841) -> (15.4824, 10.1569)
  arc A3825 (15.4824, 10.1569) -> (15.33, 10.1569) centre (15.4062, 10.1569) ccw
  line L3830 (15.3523, 9.7302) -> (15.5387, 9.5438)
  arc A3826 (15.5387, 9.5438) -> (15.6465, 9.6516) centre (15.5926, 9.5977) ccw
  line L3831 (15.6465, 9.6516) -> (15.4601, 9.838)
  arc A3827 (15.4601, 9.838) -> (15.3523, 9.7302) centre (15.4062, 9.7841) ccw
  line L3832 (15.6465, 9.5438) -> (16.3922, 10.2895)
  arc A3828 (16.3922, 10.2895) -> (16.2844, 10.3973) centre (16.3383, 10.3434) ccw
  line L3833 (16.2844, 10.3973) -> (15.5387, 9.6516)
  arc A3829 (15.5387, 9.6516) -> (15.6465, 9.5438) centre (15.5926, 9.5977) ccw
  line L3834 (16.3922, 10.7131) -> (16.5786, 10.8995)
  arc A3830 (16.5786, 10.8995) -> (16.4708, 11.0073) centre (16.5247, 10.9534) ccw
  line L3835 (16.4708, 11.0073) -> (16.2844, 10.8209)
  arc A3831 (16.2844, 10.8209) -> (16.3922, 10.7131) centre (16.3383, 10.767) ccw
  line L3836 (16.6009, 10.9534) -> (16.6009, 11.3262)
  arc A3832 (16.6009, 11.3262) -> (16.4485, 11.3262) centre (16.5247, 11.3262) ccw
  line L3837 (16.4485, 11.3262) -> (16.4485, 10.9534)
  arc A3833 (16.4485, 10.9534) -> (16.6009, 10.9534) centre (16.5247, 10.9534) ccw
  line L3838 (16.5786, 11.3801) -> (16.3922, 11.5666)
  arc A3834 (16.3922, 11.5666) -> (16.2844, 11.4588) centre (16.3383, 11.5127) ccw
  line L3839 (16.2844, 11.4588) -> (16.4708, 11.2723)
  arc A3835 (16.4708, 11.2723) -> (16.5786, 11.3801) centre (16.5247, 11.3262) ccw
  line L3840 (16.3383, 11.5889) -> (16.1519, 11.5889)
  arc A3836 (16.1519, 11.5889) -> (16.1519, 11.4365) centre (16.1519, 11.5127) ccw
  line L3841 (16.1519, 11.4365) -> (16.3383, 11.4365)
  arc A3837 (16.3383, 11.4365) -> (16.3383, 11.5889) centre (16.3383, 11.5127) ccw
  line L3842 (16.098, 11.5666) -> (15.9115, 11.3801)
  arc A3838 (15.9115, 11.3801) -> (16.0193, 11.2723) centre (15.9654, 11.3262) ccw
  line L3843 (16.0193, 11.2723) -> (16.2058, 11.4588)
  arc A3839 (16.2058, 11.4588) -> (16.098, 11.5666) centre (16.1519, 11.5127) ccw
  line L3844 (16.0193, 11.3801) -> (15.8329, 11.5666)
  arc A3840 (15.8329, 11.5666) -> (15.7251, 11.4588) centre (15.779, 11.5127) ccw
  line L3845 (15.7251, 11.4588) -> (15.9115, 11.2723)
  arc A3841 (15.9115, 11.2723) -> (16.0193, 11.3801) centre (15.9654, 11.3262) ccw
  line L3846 (15.779, 11.5889) -> (15.5926, 11.5889)
  arc A3842 (15.5926, 11.5889) -> (15.5926, 11.4365) centre (15.5926, 11.5127) ccw
  line L3847 (15.5926, 11.4365) -> (15.779, 11.4365)
  arc A3843 (15.779, 11.4365) -> (15.779, 11.5889) centre (15.779, 11.5127) ccw
  line L3848 (15.5387, 11.5666) -> (15.3523, 11.3801)
  arc A3844 (15.3523, 11.3801) -> (15.4601, 11.2723) centre (15.4062, 11.3262) ccw
  line L3849 (15.4601, 11.2723) -> (15.6465, 11.4588)
  arc A3845 (15.6465, 11.4588) -> (15.5387, 11.5666) centre (15.5926, 11.5127) ccw
  line L3850 (15.33, 11.3262) -> (15.33, 10.9534)
  arc A3846 (15.33, 10.9534) -> (15.4824, 10.9534) centre (15.4062, 10.9534) ccw
  line L3851 (15.4824, 10.9534) -> (15.4824, 11.3262)
  arc A3847 (15.4824, 11.3262) -> (15.33, 11.3262) centre (15.4062, 11.3262) ccw
  line L3852 (15.3523, 10.8995) -> (15.5387, 10.7131)
  arc A3848 (15.5387, 10.7131) -> (15.6465, 10.8209) centre (15.5926, 10.767) ccw
  line L3853 (15.6465, 10.8209) -> (15.4601, 11.0073)
  arc A3849 (15.4601, 11.0073) -> (15.3523, 10.8995) centre (15.4062, 10.9534) ccw
  line L3854 (15.5926, 10.6908) -> (15.779, 10.6908)
  arc A3850 (15.779, 10.6908) -> (15.779, 10.8432) centre (15.779, 10.767) ccw
  line L3855 (15.779, 10.8432) -> (15.5926, 10.8432)
  arc A3851 (15.5926, 10.8432) -> (15.5926, 10.6908) centre (15.5926, 10.767) ccw
  line L3856 (15.8329, 10.7131) -> (16.0193, 10.8995)
  arc A3852 (16.0193, 10.8995) -> (15.9115, 11.0073) centre (15.9654, 10.9534) ccw
  line L3857 (15.9115, 11.0073) -> (15.7251, 10.8209)
  arc A3853 (15.7251, 10.8209) -> (15.8329, 10.7131) centre (15.779, 10.767) ccw
  line L3858 (15.9115, 10.8995) -> (16.098, 10.7131)
  arc A3854 (16.098, 10.7131) -> (16.2058, 10.8209) centre (16.1519, 10.767) ccw
  line L3859 (16.2058, 10.8209) -> (16.0193, 11.0073)
  arc A3855 (16.0193, 11.0073) -> (15.9115, 10.8995) centre (15.9654, 10.9534) ccw
  line L3860 (16.1519, 10.6908) -> (16.3383, 10.6908)
  arc A3856 (16.3383, 10.6908) -> (16.3383, 10.8432) centre (16.3383, 10.767) ccw
  line L3861 (16.3383, 10.8432) -> (16.1519, 10.8432)
  arc A3857 (16.1519, 10.8432) -> (16.1519, 10.6908) centre (16.1519, 10.767) ccw
  line L3862 (16.0416, 10.9534) -> (16.0416, 11.3262)
  arc A3858 (16.0416, 11.3262) -> (15.8892, 11.3262) centre (15.9654, 11.3262) ccw
  line L3863 (15.8892, 11.3262) -> (15.8892, 10.9534)
  arc A3859 (15.8892, 10.9534) -> (16.0416, 10.9534) centre (15.9654, 10.9534) ccw
  line L3864 (15.4062, 11.8601) -> (16.5247, 11.8601)
  arc A3860 (16.5247, 11.8601) -> (16.5247, 12.0125) centre (16.5247, 11.9363) ccw
  line L3865 (16.5247, 12.0125) -> (15.4062, 12.0125)
  arc A3861 (15.4062, 12.0125) -> (15.4062, 11.8601) centre (15.4062, 11.9363) ccw
  line L3866 (16.5786, 11.9902) -> (16.2058, 12.363)
  arc A3862 (16.2058, 12.363) -> (16.098, 12.2552) centre (16.1519, 12.3091) ccw
  line L3867 (16.098, 12.2552) -> (16.4708, 11.8824)
  arc A3863 (16.4708, 11.8824) -> (16.5786, 11.9902) centre (16.5247, 11.9363) ccw
  line L3868 (16.2058, 12.2552) -> (16.5786, 12.6281)
  arc A3864 (16.5786, 12.6281) -> (16.4708, 12.7359) centre (16.5247, 12.682) ccw
  line L3869 (16.4708, 12.7359) -> (16.098, 12.363)
  arc A3865 (16.098, 12.363) -> (16.2058, 12.2552) centre (16.1519, 12.3091) ccw
  line L3870 (16.5247, 12.7582) -> (15.4062, 12.7582)
  arc A3866 (15.4062, 12.7582) -> (15.4062, 12.6058) centre (15.4062, 12.682) ccw
  line L3871 (15.4062, 12.6058) -> (16.5247, 12.6058)
  arc A3867 (16.5247, 12.6058) -> (16.5247, 12.7582) centre (16.5247, 12.682) ccw
  line L3872 (15.4062, 13.0294) -> (16.5247, 13.0294)
  arc A3868 (16.5247, 13.0294) -> (16.5247, 13.1818) centre (16.5247, 13.1056) ccw
  line L3873 (16.5247, 13.1818) -> (15.4062, 13.1818)
  arc A3869 (15.4062, 13.1818) -> (15.4062, 13.0294) centre (15.4062, 13.1056) ccw
  line L3874 (16.5786, 13.1595) -> (16.2058, 13.5323)
  arc A3870 (16.2058, 13.5323) -> (16.098, 13.4245) centre (16.1519, 13.4784) ccw
  line L3875 (16.098, 13.4245) -> (16.4708, 13.0517)
  arc A3871 (16.4708, 13.0517) -> (16.5786, 13.1595) centre (16.5247, 13.1056) ccw
  line L3876 (16.2058, 13.4245) -> (16.5786, 13.7974)
  arc A3872 (16.5786, 13.7974) -> (16.4708, 13.9052) centre (16.5247, 13.8513) ccw
  line L3877 (16.4708, 13.9052) -> (16.098, 13.5323)
  arc A3873 (16.098, 13.5323) -> (16.2058, 13.4245) centre (16.1519, 13.4784) ccw
  line L3878 (16.5247, 13.9275) -> (15.4062, 13.9275)
  arc A3874 (15.4062, 13.9275) -> (15.4062, 13.7751) centre (15.4062, 13.8513) ccw
  line L3879 (15.4062, 13.7751) -> (16.5247, 13.7751)
  arc A3875 (16.5247, 13.7751) -> (16.5247, 13.9275) centre (16.5247, 13.8513) ccw
  line L3880 (15.4062, 15.7408) -> (16.5247, 15.7408)
  arc A3876 (16.5247, 15.7408) -> (16.5247, 15.8932) centre (16.5247, 15.817) ccw
  line L3881 (16.5247, 15.8932) -> (15.4062, 15.8932)
  arc A3877 (15.4062, 15.8932) -> (15.4062, 15.7408) centre (15.4062, 15.817) ccw
  line L3882 (16.6009, 15.4442) -> (16.6009, 16.1899)
  arc A3878 (16.6009, 16.1899) -> (16.4485, 16.1899) centre (16.5247, 16.1899) ccw
  line L3883 (16.4485, 16.1899) -> (16.4485, 15.4442)
  arc A3879 (16.4485, 15.4442) -> (16.6009, 15.4442) centre (16.5247, 15.4442) ccw
  line L3884 (15.4062, 16.5373) -> (16.5247, 16.5373)
  arc A3880 (16.5247, 16.5373) -> (16.5247, 16.6897) centre (16.5247, 16.6135) ccw
  line L3885 (16.5247, 16.6897) -> (15.4062, 16.6897)
  arc A3881 (15.4062, 16.6897) -> (15.4062, 16.5373) centre (15.4062, 16.6135) ccw
  line L3886 (16.6009, 16.6135) -> (16.6009, 17.1727)
  arc A3882 (16.6009, 17.1727) -> (16.4485, 17.1727) centre (16.5247, 17.1727) ccw
  line L3887 (16.4485, 17.1727) -> (16.4485, 16.6135)
  arc A3883 (16.4485, 16.6135) -> (16.6009, 16.6135) centre (16.5247, 16.6135) ccw
  line L3888 (16.5786, 17.2266) -> (16.3922, 17.4131)
  arc A3884 (16.3922, 17.4131) -> (16.2844, 17.3053) centre (16.3383, 17.3592) ccw
  line L3889 (16.2844, 17.3053) -> (16.4708, 17.1188)
  arc A3885 (16.4708, 17.1188) -> (16.5786, 17.2266) centre (16.5247, 17.1727) ccw
  line L3890 (16.3383, 17.4354) -> (15.9654, 17.4354)
  arc A3886 (15.9654, 17.4354) -> (15.9654, 17.283) centre (15.9654, 17.3592) ccw
  line L3891 (15.9654, 17.283) -> (16.3383, 17.283)
  arc A3887 (16.3383, 17.283) -> (16.3383, 17.4354) centre (16.3383, 17.3592) ccw
  line L3892 (15.9115, 17.4131) -> (15.7251, 17.2266)
  arc A3888 (15.7251, 17.2266) -> (15.8329, 17.1188) centre (15.779, 17.1727) ccw
  line L3893 (15.8329, 17.1188) -> (16.0193, 17.3053)
  arc A3889 (16.0193, 17.3053) -> (15.9115, 17.4131) centre (15.9654, 17.3592) ccw
  line L3894 (15.7028, 17.1727) -> (15.7028, 16.6135)
  arc A3890 (15.7028, 16.6135) -> (15.8552, 16.6135) centre (15.779, 16.6135) ccw
  line L3895 (15.8552, 16.6135) -> (15.8552, 17.1727)
  arc A3891 (15.8552, 17.1727) -> (15.7028, 17.1727) centre (15.779, 17.1727) ccw
  line L3896 (15.8329, 17.0402) -> (15.4601, 17.4131)
  arc A3892 (15.4601, 17.4131) -> (15.3523, 17.3053) centre (15.4062, 17.3592) ccw
  line L3897 (15.3523, 17.3053) -> (15.7251, 16.9324)
  arc A3893 (15.7251, 16.9324) -> (15.8329, 17.0402) centre (15.779, 16.9863) ccw
  line L3898 (15.4062, 17.7066) -> (16.1519, 17.7066)
  arc A3894 (16.1519, 17.7066) -> (16.1519, 17.859) centre (16.1519, 17.7828) ccw
  line L3899 (16.1519, 17.859) -> (15.4062, 17.859)
  arc A3895 (15.4062, 17.859) -> (15.4062, 17.7066) centre (15.4062, 17.7828) ccw
  line L3900 (16.2058, 17.7289) -> (16.5786, 18.1017)
  arc A3896 (16.5786, 18.1017) -> (16.4708, 18.2095) centre (16.5247, 18.1556) ccw
  line L3901 (16.4708, 18.2095) -> (16.098, 17.8367)
  arc A3897 (16.098, 17.8367) -> (16.2058, 17.7289) centre (16.1519, 17.7828) ccw
  line L3902 (16.5786, 18.2095) -> (16.2058, 18.5824)
  arc A3898 (16.2058, 18.5824) -> (16.098, 18.4746) centre (16.1519, 18.5285) ccw
  line L3903 (16.098, 18.4746) -> (16.4708, 18.1017)
  arc A3899 (16.4708, 18.1017) -> (16.5786, 18.2095) centre (16.5247, 18.1556) ccw
  line L3904 (16.1519, 18.6047) -> (15.4062, 18.6047)
  arc A3900 (15.4062, 18.6047) -> (15.4062, 18.4523) centre (15.4062, 18.5285) ccw
  line L3905 (15.4062, 18.4523) -> (16.1519, 18.4523)
  arc A3901 (16.1519, 18.4523) -> (16.1519, 18.6047) centre (16.1519, 18.5285) ccw
  line L3906 (16.0416, 17.7828) -> (16.0416, 18.5285)
  arc A3902 (16.0416, 18.5285) -> (15.8892, 18.5285) centre (15.9654, 18.5285) ccw
  line L3907 (15.8892, 18.5285) -> (15.8892, 17.7828)
  arc A3903 (15.8892, 17.7828) -> (16.0416, 17.7828) centre (15.9654, 17.7828) ccw
  line L3908 (15.4062, 18.8759) -> (16.5247, 18.8759)
  arc A3904 (16.5247, 18.8759) -> (16.5247, 19.0283) centre (16.5247, 18.9521) ccw
  line L3909 (16.5247, 19.0283) -> (15.4062, 19.0283)
  arc A3905 (15.4062, 19.0283) -> (15.4062, 18.8759) centre (15.4062, 18.9521) ccw
  line L3910 (16.567, 19.0155) -> (15.4485, 19.7612)
  arc A3906 (15.4485, 19.7612) -> (15.3639, 19.6344) centre (15.4062, 19.6978) ccw
  line L3911 (15.3639, 19.6344) -> (16.4824, 18.8887)
  arc A3907 (16.4824, 18.8887) -> (16.567, 19.0155) centre (16.5247, 18.9521) ccw
  line L3912 (15.4062, 19.6216) -> (16.5247, 19.6216)
  arc A3908 (16.5247, 19.6216) -> (16.5247, 19.774) centre (16.5247, 19.6978) ccw
  line L3913 (16.5247, 19.774) -> (15.4062, 19.774)
  arc A3909 (15.4062, 19.774) -> (15.4062, 19.6216) centre (15.4062, 19.6978) ccw
  line L3914 (16.2844, 20.8132) -> (16.4708, 20.6267)
  arc A3910 (16.4708, 20.6267) -> (16.5786, 20.7345) centre (16.5247, 20.6806) ccw
  line L3915 (16.5786, 20.7345) -> (16.3922, 20.921)
  arc A3911 (16.3922, 20.921) -> (16.2844, 20.8132) centre (16.3383, 20.8671) ccw
  line L3916 (16.4485, 20.6806) -> (16.4485, 20.3078)
  arc A3912 (16.4485, 20.3078) -> (16.6009, 20.3078) centre (16.5247, 20.3078) ccw
  line L3917 (16.6009, 20.3078) -> (16.6009, 20.6806)
  arc A3913 (16.6009, 20.6806) -> (16.4485, 20.6806) centre (16.5247, 20.6806) ccw
  line L3918 (16.4708, 20.3617) -> (16.2844, 20.1753)
  arc A3914 (16.2844, 20.1753) -> (16.3922, 20.0675) centre (16.3383, 20.1214) ccw
  line L3919 (16.3922, 20.0675) -> (16.5786, 20.2539)
  arc A3915 (16.5786, 20.2539) -> (16.4708, 20.3617) centre (16.5247, 20.3078) ccw
  line L3920 (16.3383, 20.1976) -> (16.1519, 20.1976)
  arc A3916 (16.1519, 20.1976) -> (16.1519, 20.0452) centre (16.1519, 20.1214) ccw
  line L3921 (16.1519, 20.0452) -> (16.3383, 20.0452)
  arc A3917 (16.3383, 20.0452) -> (16.3383, 20.1976) centre (16.3383, 20.1214) ccw
  line L3922 (16.2058, 20.1753) -> (16.0193, 20.3617)
  arc A3918 (16.0193, 20.3617) -> (15.9115, 20.2539) centre (15.9654, 20.3078) ccw
  line L3923 (15.9115, 20.2539) -> (16.098, 20.0675)
  arc A3919 (16.098, 20.0675) -> (16.2058, 20.1753) centre (16.1519, 20.1214) ccw
  line L3924 (16.0416, 20.3078) -> (16.0416, 20.6806)
  arc A3920 (16.0416, 20.6806) -> (15.8892, 20.6806) centre (15.9654, 20.6806) ccw
  line L3925 (15.8892, 20.6806) -> (15.8892, 20.3078)
  arc A3921 (15.8892, 20.3078) -> (16.0416, 20.3078) centre (15.9654, 20.3078) ccw
  line L3926 (16.0193, 20.7345) -> (15.8329, 20.921)
  arc A3922 (15.8329, 20.921) -> (15.7251, 20.8132) centre (15.779, 20.8671) ccw
  line L3927 (15.7251, 20.8132) -> (15.9115, 20.6267)
  arc A3923 (15.9115, 20.6267) -> (16.0193, 20.7345) centre (15.9654, 20.6806) ccw
  line L3928 (15.779, 20.9433) -> (15.5926, 20.9433)
  arc A3924 (15.5926, 20.9433) -> (15.5926, 20.7909) centre (15.5926, 20.8671) ccw
  line L3929 (15.5926, 20.7909) -> (15.779, 20.7909)
  arc A3925 (15.779, 20.7909) -> (15.779, 20.9433) centre (15.779, 20.8671) ccw
  line L3930 (15.5387, 20.921) -> (15.3523, 20.7345)
  arc A3926 (15.3523, 20.7345) -> (15.4601, 20.6267) centre (15.4062, 20.6806) ccw
  line L3931 (15.4601, 20.6267) -> (15.6465, 20.8132)
  arc A3927 (15.6465, 20.8132) -> (15.5387, 20.921) centre (15.5926, 20.8671) ccw
  line L3932 (15.33, 20.6806) -> (15.33, 20.3078)
  arc A3928 (15.33, 20.3078) -> (15.4824, 20.3078) centre (15.4062, 20.3078) ccw
  line L3933 (15.4824, 20.3078) -> (15.4824, 20.6806)
  arc A3929 (15.4824, 20.6806) -> (15.33, 20.6806) centre (15.4062, 20.6806) ccw
  line L3934 (15.3523, 20.2539) -> (15.5387, 20.0675)
  arc A3930 (15.5387, 20.0675) -> (15.6465, 20.1753) centre (15.5926, 20.1214) ccw
  line L3935 (15.6465, 20.1753) -> (15.4601, 20.3617)
  arc A3931 (15.4601, 20.3617) -> (15.3523, 20.2539) centre (15.4062, 20.3078) ccw
  line L3936 (15.4824, 21.2907) -> (15.4824, 21.6635)
  arc A3932 (15.4824, 21.6635) -> (15.33, 21.6635) centre (15.4062, 21.6635) ccw
  line L3937 (15.33, 21.6635) -> (15.33, 21.2907)
  arc A3933 (15.33, 21.2907) -> (15.4824, 21.2907) centre (15.4062, 21.2907) ccw
  line L3938 (15.4062, 21.4009) -> (16.5247, 21.4009)
  arc A3934 (16.5247, 21.4009) -> (16.5247, 21.5533) centre (16.5247, 21.4771) ccw
  line L3939 (16.5247, 21.5533) -> (15.4062, 21.5533)
  arc A3935 (15.4062, 21.5533) -> (15.4062, 21.4009) centre (15.4062, 21.4771) ccw
  line L3940 (16.6009, 21.2907) -> (16.6009, 21.6635)
  arc A3936 (16.6009, 21.6635) -> (16.4485, 21.6635) centre (16.5247, 21.6635) ccw
  line L3941 (16.4485, 21.6635) -> (16.4485, 21.2907)
  arc A3937 (16.4485, 21.2907) -> (16.6009, 21.2907) centre (16.5247, 21.2907) ccw
  line L3942 (15.4062, 22.3668) -> (16.5247, 22.3668)